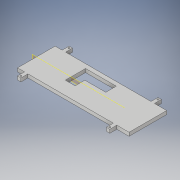
# Autodesk Inventor part: BackPanel
Saved by Autodesk Inventor 2018 (Build 220112000, 112)
## iProperties
Created: 2018-10-20
Part Number: BackPanel
Material: Generic
Document SubType Name: Modeling
Designer: jpark
Density: 1 g/cm^3
Appearance: Default
Author: jpark
Autodesk Inventor part; units mm, degrees
ref_plane "YZ Plane" through (0, 0, 0) normal (1, 0, 0) x (0, 1, 0)
ref_plane "XZ Plane" through (0, 0, 0) normal (0, 1, 0) x (-1, 0, 0)
ref_plane "XY Plane" through (0, 0, 0) normal (0, 0, 1) x (1, 0, 0)
sketch "Sketch1" plane through (0, 0, 0) normal (0, 1, 0) x (-1, 0, 0)
  line L0 (0, 0) -> (203.2, 0)
  line L1 (203.2, 0) -> (203.2, -68.58)
  line L2 (203.2, -68.58) -> (0, -68.58)
  line L3 (0, -68.58) -> (0, 0)
  dimension "d0" = 203.2
  dimension "d1" = 68.58
  constraints: 8 end point, 2 parallel, 1 horizontal, 1 perpendicular
  measures "d0" distance of L1.end L2.end
  measures "d1" distance of L0.end L1.end
extrude "Extrusion1" add sketch "Sketch1" along normal blind 6.35
sketch "Sketch2" plane through (0, 6.35, 0) normal (0, 1, 0) x (1, 0, 0)
  line L0 (-184.15, 0) -> (-190.5, 0)
  line L1 (-190.5, 0) -> (-190.5, -12.7)
  line L2 (-190.5, -12.7) -> (-184.15, -12.7)
  line L3 (-184.15, -12.7) -> (-184.15, 0)
  circle A0 centre (-187.325, -9.525) radius 1.397
  line L4 (-203.2, 0) -> (0, 0) projected
  line L5 (-22.225, 0) -> (-28.575, 0)
  line L6 (-28.575, 0) -> (-28.575, -12.7)
  line L7 (-28.575, -12.7) -> (-22.225, -12.7)
  line L8 (-22.225, -12.7) -> (-22.225, 0)
  circle A1 centre (-25.4, -9.525) radius 1.397
  dimension "d4" = 12.7
  dimension "d5" = 6.35
  dimension "d6" = 2.794
  dimension "d7" = 3.175
  dimension "d8" = 3.175
  dimension "d9" = 0
  dimension "d10" = 12.7
  dimension "d11" = 12.7
  dimension "d12" = 6.35
  dimension "d13" = 2.794
  dimension "d14" = 3.175
  dimension "d15" = 3.175
  dimension "d16" = 0
  dimension "d20" = 25.4
  constraints: 16 end point, 4 parallel, 2 centre point, 2 horizontal, 2 perpendicular
  measures "d4" distance of L0.end L1.end
  measures "d5" distance of L1.end L2.end
  measures "d6" diameter of A0
  measures "d7" distance from line of L2 A0.centre
  measures "d8" distance from line of L3 A0.centre
  measures "d9" distance between parallel lines of L4 L0
  measures "d10" distance from line of L4.start L1
  measures "d11" distance of L5.end L6.end
  measures "d12" distance of L6.end L7.end
  measures "d13" diameter of A1
  measures "d14" distance from line of L7 A1.centre
  measures "d15" distance from line of L8 A1.centre
  measures "d16" distance between parallel lines of L4 L5
  measures "d20" horizontal distance of L4.end A1.centre
extrude "Extrusion2" add sketch "Sketch2" against normal blind 6.35
ref_plane "Work Plane1" through (-184.15, 0, -34.29) normal (0, 0, 1) x (1, 0, 0)
mirror "Mirror1" about plane through (-184.15, 0, -34.29) normal (0, 0, 1) of "Extrusion2"
sketch "Sketch3" plane through (0, 6.35, 0) normal (0, 1, 0) x (1, 0, 0)
  line L0 (-140.1724, 41.91) -> (-84.2924, 41.91)
  line L1 (-84.2924, 41.91) -> (-84.2924, 60.96)
  line L2 (-84.2924, 60.96) -> (-140.1724, 60.96)
  line L3 (-140.1724, 60.96) -> (-140.1724, 41.91)
  line L4 (-140.1724, 41.91) -> (-122.3924, 41.91)
  line L5 (-122.3924, 41.91) -> (-122.3924, 24.13)
  line L6 (-122.3924, 24.13) -> (-140.1724, 24.13)
  line L7 (-140.1724, 24.13) -> (-140.1724, 41.91)
  line L8 (-28.575, 68.58) -> (-184.15, 68.58) projected
  point P0 (0, 0)
  dimension "d21" = 19.05
  dimension "d22" = 55.88
  dimension "d23" = 17.78
  dimension "d24" = 17.78
  dimension "d25" = 7.62
  constraints: 16 end point, 4 parallel, 2 horizontal, 2 perpendicular
  measures "d21" distance of L0.end L1.end
  measures "d22" distance of L0.start L0.end
  measures "d23" distance of L4.end L5.end
  measures "d24" distance of L5.end L6.end
  measures "d25" distance between parallel lines of L8 L2
extrude "Extrusion3" cut sketch "Sketch3" against normal blind 25.4
body "Solid1"
